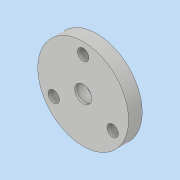
# Autodesk Inventor part: spoolPinionBearingHolder
Saved by Autodesk Inventor 2017 (Build 210142000, 142)
## iProperties
Created: 2016-11-06
Part Number: spoolPinionBearingHolder
Material: Generic
Document SubType Name: Modeling
Designer: techn
Density: 1 g/cm^3
Appearance: Default
Author: techn
Autodesk Inventor part; units mm, degrees
ref_plane "YZ Plane" through (0, 0, 0) normal (1, 0, 0) x (0, 1, 0)
ref_plane "XZ Plane" through (0, 0, 0) normal (0, 1, 0) x (-1, 0, 0)
ref_plane "XY Plane" through (0, 0, 0) normal (0, 0, 1) x (1, 0, 0)
sketch "Sketch1" plane through (0, 0, 0) normal (0, 0, 1) x (1, 0, 0)
  circle A0 centre (0, 0) radius 3.175
  line L0 (0, 0) -> (0, 9.525)
  circle A1 centre (0, 9.525) radius 1.5875
  circle A2 centre (-8.2489, -4.7625) radius 1.5875
  circle A3 centre (8.2489, -4.7625) radius 1.5875
  circle A4 centre (0, 0) radius 12.7
  dimension "d0" = 6.35
  dimension "d1" = 9.525
  dimension "d2" = 3.175
  dimension "d5" = 360
  dimension "d7" = 25.4
  constraints: 5 centre point, 3 coincident, 2 end point, 1 vertical, 7 other
  measures "d0" diameter of A0
  measures "d1" distance of L0.start L0.end
  measures "d2" diameter of A1
  measures "d7" diameter of A4
extrude "Extrusion1" add sketch "Sketch1" along normal blind 3.175
sketch "Sketch2" plane through (0, 0, 3.175) normal (0, 0, 1) x (1, 0, 0)
  circle A0 centre (0, 0) radius 3.175 projected
  circle A1 centre (8.2489, -4.7625) radius 1.5875 projected
  circle A2 centre (-8.2489, -4.7625) radius 1.5875 projected
  circle A3 centre (0, 9.525) radius 1.5875 projected
  circle A4 centre (0, 0) radius 12.7 projected
  circle A5 centre (0, 0) radius 2.3813
  dimension "d10" = 4.7625
  constraints: 1 centre point, 1 coincident
  measures "d10" diameter of A5
extrude "Extrusion2" add sketch "Sketch2" along normal blind 0.635 contours A0 | A4
body "Solid1"
